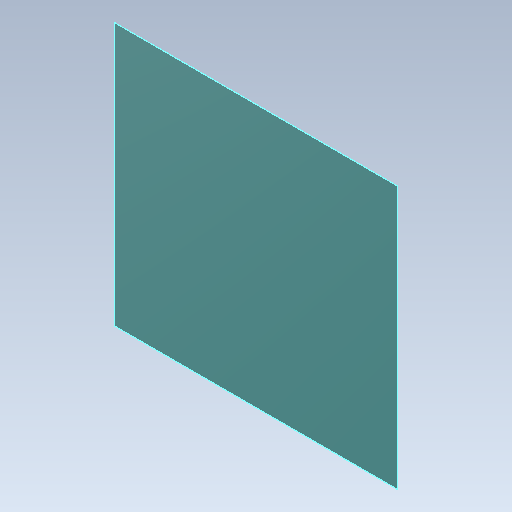
# Autodesk Inventor part: JST
Saved by Autodesk Inventor 2021 (Build 250183000, 183)
## iProperties
Created: 2020-11-03
Part Number: JST
Material: Generic
Document SubType Name: Modeling
Designer: faiya
Density: 1 g/cm^3
Appearance: JSTPH2, JST
Author: faiya
Autodesk Inventor part; units mm, degrees
ref_plane "YZ Plane" through (0, 0, 0) normal (1, 0, 0) x (0, 1, 0)
ref_plane "XZ Plane" through (0, 0, 0) normal (0, 1, 0) x (-1, 0, 0)
ref_plane "XY Plane" through (0, 0, 0) normal (0, 0, 1) x (1, 0, 0)
sketch "JSTPH2, JST_3" plane through (0, 0, 0) normal (0, 0, 1) x (1, 0, 0)
  line L0 (-4.1016, 3.1016) -> (4.1016, 3.1016)
  line L1 (4.1016, 3.1016) -> (4.1016, -4.5)
  line L2 (4.1016, -4.5) -> (-4.1016, -4.5)
  line L3 (-4.1016, -4.5) -> (-4.1016, 3.1016)
  constraints: 8 end point
extrude "Extrusion1" add sketch "JSTPH2, JST_3" along normal blind 0.01
body "Solid1"
